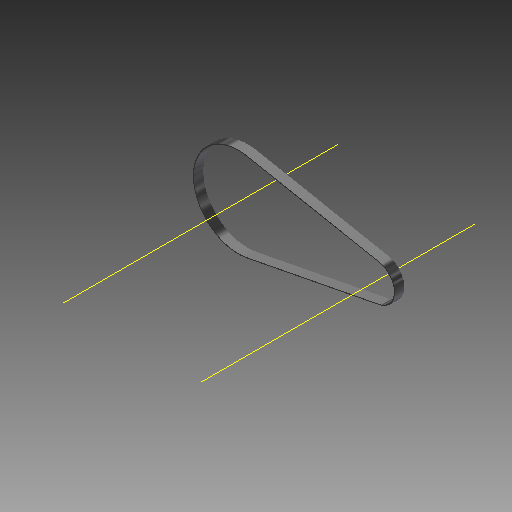
# Autodesk Inventor part: Synchronous Belt
Saved by Autodesk Inventor 2019 (Build 230136000, 136)
## iProperties
Created: 2019-10-19
Part Number: Synchronous Belt
Material: Rubber
Document SubType Name: Modeling
Designer: admin
Density: 1 g/cm^3
Appearance: Rubber - Black - Version 1.1
CustomPartVersion: 1
d6: 0.000 mm
d8: 0.000 mm
d9: 0.000 mm
d10: 0.000 mm
d11: 0.000 mm
Author: admin
Autodesk Inventor part; units mm, degrees
sketch "Sketch Path" plane through (0, 0, 0) normal (0, 0, 1) x (1, 0, 0)
  arc A0 (3.793, -19.5294) -> (3.793, 19.5294) centre (0, 0) ccw
  arc A1 (-136.9837, 46.8707) -> (-136.9837, -46.8707) centre (-146.0868, 0) ccw
  line L0 (-136.9837, 46.8707) -> (3.793, 19.5294)
  line L1 (3.793, -19.5294) -> (-136.9837, -46.8707)
  constraints: 4 end point, 2 point on circle, 1 centre point, 1 vertical alignment, 2 other
ref_plane "Cross Section Plane" through (3.793, 19.5294, 0) normal (-0.9817, 0.1907, 0) x (0, 0, 1)
ref_plane "Work Plane2" through (0, 0, 0) normal (-1, 0, 0) x (0, 0, 1)
ref_plane "Work Plane3" through (-146.0868, 0, 0) normal (0.9914, 0.1305, 0) x (0, 0, 1)
sketch "Cross Section" plane through (3.793, 19.5294, 0) normal (-0.9817, 0.1907, 0) x (0, 0, 1)
  line L0 (-5, 0.5) -> (5, 0.5)
  line L1 (5, 0.5) -> (5, -0.5)
  line L2 (5, -0.5) -> (-5, -0.5)
  line L3 (-5, -0.5) -> (-5, 0.5)
  line L4 (-5, 0) -> (5, 0) construction
  point P0 (0, 0)
  point P1 (0, 0)
  dimension "d0" = 10
  dimension "d4" = 0.5
  dimension "d5" = 0.5
  constraints: 10 end point, 3 midpoint, 2 parallel, 1 coincident, 1 horizontal, 1 perpendicular, 1 other
  measures "d0" distance between parallel lines of L1 L3
  measures "d4" distance between parallel lines of L2 L4
  measures "d5" distance between parallel lines of L4 L0
sweep "Belt" add profiles "Cross Section" path "Sketch Path"
equation "\"d0\" = da_B"
equation "\"d4\" = da_a"
equation "\"d5\" = da_a2"
equation "\"da_B\" = 10"
equation "\"da_pb\" = 5"
equation "\"da_a\" = 0.5"
equation "\"da_S\" = 2.65"
equation "\"da_Beta\" = 20deg"
equation "\"da_Ht\" = 1.2"
equation "\"da_H\" = 2.2"
equation "\"da_a2\" = 0.5"
body "Solid1"
